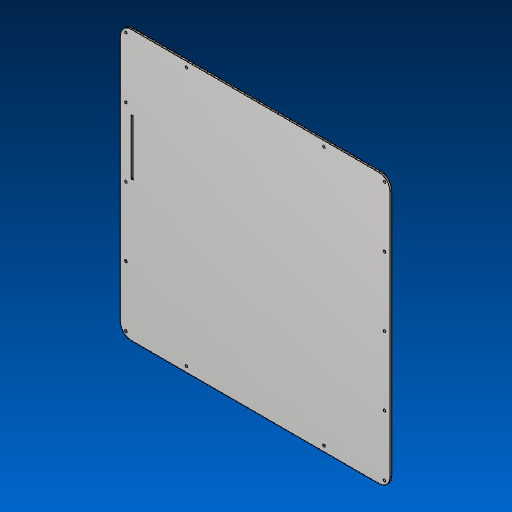
# Autodesk Inventor part: left_panel
Saved by Autodesk Inventor 2018 (Build 220112000, 112)
## iProperties
Created: 2019-10-14
Part Number: left_panel
Material: アルミニウム 6061
Document SubType Name: Modeling
Designer: gisen
Density: 2.7 g/cm^3
Appearance: アルミニウム - フラット
Author: gisen
Autodesk Inventor part; units mm, degrees
ref_plane "YZ Plane" through (0, 0, 0) normal (1, 0, 0) x (0, 1, 0)
ref_plane "XZ Plane" through (0, 0, 0) normal (0, 1, 0) x (-1, 0, 0)
ref_plane "XY Plane" through (0, 0, 0) normal (0, 0, 1) x (1, 0, 0)
sketch "スケッチ1" plane through (0, 0, 0) normal (0, 0, 1) x (1, 0, 0)
  line L0 (-225, -245) -> (225, -245)
  line L1 (245, -225) -> (245, 225)
  line L2 (225, 245) -> (-225, 245)
  line L3 (-245, 225) -> (-245, -225)
  line L4 (-245, -245) -> (245, 245) construction
  line L5 (245, -245) -> (-245, 245) construction
  circle A0 centre (-235, 235) radius 2.25
  circle A1 centre (235, 235) radius 2.25
  circle A2 centre (-235, -235) radius 2.25
  circle A3 centre (235, -235) radius 2.25
  arc A4 (-225, 245) -> (-245, 225) centre (-225, 225) ccw
  arc A5 (245, 225) -> (225, 245) centre (225, 225) ccw
  arc A6 (225, -245) -> (245, -225) centre (225, -225) ccw
  arc A7 (-245, -225) -> (-225, -245) centre (-225, -225) ccw
  point P0 (0, 0)
  dimension "d0" = 490
  dimension "d1" = 490
  dimension "d2" = 4.5
  dimension "d3" = 10
  dimension "d4" = 10
  dimension "d5" = 10
  dimension "d6" = 10
  dimension "d7" = 10
  dimension "d8" = 10
  dimension "d9" = 10
  dimension "d10" = 10
  dimension "d11" = 20
  constraints: 12 end point, 8 centre point, 8 point on circle, 8 point on line, 8 tangent, 6 equal radius, 2 midpoint, 2 parallel, 1 horizontal, 1 perpendicular
  measures "d0" distance of L5.end L4.end
  measures "d1" distance of L4.end L5.start
  measures "d2" diameter of A0
  measures "d3" distance from line of A0.centre L2
  measures "d4" distance from line of L3 A0.centre
  measures "d5" distance from line of A1.centre L2
  measures "d6" distance from line of L1 A1.centre
  measures "d7" distance from line of L1 A3.centre
  measures "d8" distance from line of L0 A3.centre
  measures "d9" distance from line of L0 A2.centre
  measures "d10" distance from line of L3 A2.centre
  measures "d11" radius of A4
extrude "押し出し1" add sketch "スケッチ1" along normal blind 3
sketch "スケッチ2" plane through (0, 0, 3) normal (0, 0, 1) x (1, 0, 0)
  circle A0 centre (-235, -235) radius 2.25 construction
  circle A1 centre (-235, -125) radius 2.25
  line L0 (-245, 225) -> (-245, -225) projected
  point P0 (0, 0)
  dimension "d14" = 110
  dimension "d15" = 10
  constraints: 1 centre point, 1 equal radius
  measures "d14" distance of A1.centre A0.centre
  measures "d15" distance from line of A1.centre L0
extrude "押し出し2" cut sketch "スケッチ2" against normal blind 10
sketch "スケッチ3" plane through (0, 0, 3) normal (0, 0, 1) x (1, 0, 0)
  line L0 (-225, 120.4005) -> (-222, 120.4005) construction
  line L1 (-225, 10) -> (-225, 120.4005) construction
  line L2 (-225, 10) -> (-222, 10) construction
  line L3 (-225.2, 110.0184) -> (-221.8, 110.0184)
  line L4 (-221.8, 110.0184) -> (-221.8, 9.8)
  line L5 (-221.8, 9.8) -> (-225.2, 9.8)
  line L6 (-225.2, 9.8) -> (-225.2, 110.0184)
  line L7 (-222, 120.4005) -> (-222, 10) projected
  point P0 (0, 0)
  point P1 (-222, -194.664)
  dimension "d18" = 0.2
  constraints: 8 end point, 1 other
  measures "d18" distance between parallel lines of L1 L6
extrude "押し出し3" cut sketch "スケッチ3" against normal up to surface (3 mm away)
sketch "スケッチ4" plane through (0, 0, 3) normal (0, 0, 1) x (1, 0, 0)
  circle A0 centre (-235, -235) radius 2.25 construction
  circle A1 centre (-235, -125) radius 2.25 construction
  circle A2 centre (235, -235) radius 2.25 construction
  circle A3 centre (-235, 235) radius 2.25 construction
  circle A4 centre (235, 235) radius 2.25 construction
  circle A5 centre (-235, -235) radius 2.25 construction
  circle A6 centre (-235, -125) radius 2.25 construction
  circle A7 centre (-235, -235) radius 110 construction
  circle A8 centre (-235, 235) radius 2.25 construction
  circle A9 centre (-235, 235) radius 110 construction
  circle A10 centre (235, 235) radius 110 construction
  circle A11 centre (235, -235) radius 110 construction
  line L0 (-235, -235) -> (235, -235) construction
  line L1 (235, -235) -> (235, 235) construction
  line L2 (235, 235) -> (-235, 235) construction
  line L3 (-235, 235) -> (-235, -235) construction
  line L4 (-235, 0) -> (235, 0) construction
  circle A12 centre (-235, 125) radius 2.25
  circle A13 centre (-235, 0) radius 2.25
  circle A14 centre (-125, -235) radius 2.25
  circle A15 centre (125, -235) radius 2.25
  circle A16 centre (235, -125) radius 2.25
  circle A17 centre (235, 125) radius 2.25
  circle A18 centre (125, 235) radius 2.25
  circle A19 centre (-125, 235) radius 2.25
  circle A20 centre (235, 0) radius 2.25
  point P0 (0, 0)
  constraints: 13 centre point, 12 equal radius, 10 end point, 8 point on circle, 7 point on line, 6 coincident, 2 midpoint, 2 parallel, 1 horizontal, 1 perpendicular
extrude "押し出し4" cut sketch "スケッチ4" against normal up to surface (3 mm away)
equation "\"d5\" = d3"
equation "\"d6\" = d4"
equation "\"d7\" = d6"
equation "\"d8\" = d5"
equation "\"d9\" = d8"
equation "\"d10\" = d7"
